spessorialtifrigopiccolibosch (Autodesk Fusion 360 design; units mm, degrees)
Autodesk Fusion 360 part; units mm, degrees
sketch "Sketch2" plane through (0, 0, 0) normal (0, 0, 1) x (1, 0, 0)
  line L0 (8, -13) -> (-8, -13)
  line L1 (-8, -13) -> (-8, 13)
  line L2 (-8, 13) -> (8, 13)
  line L3 (8, 13) -> (8, -13)
  line L4 (8, -13) -> (-8, 13) construction
  line L5 (-8, -13) -> (8, 13) construction
  line L6 (3, -5.5) -> (-3, -5.5)
  line L7 (-3, -5.5) -> (-3, 5.5)
  line L8 (-3, 5.5) -> (3, 5.5)
  line L9 (3, 5.5) -> (3, -5.5)
  line L10 (3, -5.5) -> (-3, 5.5) construction
  line L11 (-3, -5.5) -> (3, 5.5) construction
  dimension "d23" = 16
  dimension "d24" = 26
  dimension "d25" = 6
  dimension "d26" = 11
  constraint horizontal L0
  constraint perpendicular L0 L1
  constraint parallel L0 L2
  constraint parallel L1 L3
  constraint coincident L4 origin
  constraint coincident L5 origin
  constraint horizontal L6
  constraint perpendicular L6 L7
  constraint parallel L6 L8
  constraint parallel L7 L9
  constraint coincident L10 origin
  constraint coincident L11 origin
  measures "d23" distance of L1.end L2.end
  measures "d24" distance of L0.end L1.end
  measures "d25" distance of L7.end L8.end
  measures "d26" distance of L6.end L7.end
extrude "Extrude2" add sketch "Sketch2" along normal blind 3
fillet "Fillet6" radius 2 4 edges at (8, 13, 1.5) (-8, 13, 1.5) (-8, -13, 1.5) (8, -13, 1.5)
fillet "Fillet7" radius 2.25 4 edges at (-3, 5.5, 1.5) (3, 5.5, 1.5) (3, -5.5, 1.5) (-3, -5.5, 1.5)
extrude "Extrude1" [suppressed]
fillet "Fillet1" [suppressed]
fillet "Fillet2" [suppressed]
fillet "Fillet3" [suppressed]
fillet "Fillet4" [suppressed]
fillet "Fillet5" [suppressed]
